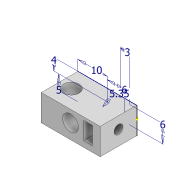
# Autodesk Inventor part: CentralStabalizerShaft
Saved by Autodesk Inventor 2022 (Build 260153000, 153)
## iProperties
Created: 2022-10-26
Part Number: CentralStabalizerShaft
Material: Generic
Document SubType Name: Modeling
Designer: MVeszpremi
Density: 1 g/cm^3
Appearance: Default
Author: MVeszpremi
Autodesk Inventor part; units mm, degrees
ref_plane "YZ Plane" through (0, 0, 0) normal (1, 0, 0) x (0, 1, 0)
ref_plane "XZ Plane" through (0, 0, 0) normal (0, 1, 0) x (-1, 0, 0)
ref_plane "XY Plane" through (0, 0, 0) normal (0, 0, 1) x (1, 0, 0)
sketch "Sketch1" plane through (0, 0, 0) normal (0, 0, 1) x (1, 0, 0)
  circle A0 centre (0, 0) radius 2.675
  line L0 (-10, 4) -> (10.0805, 4)
  line L1 (10.0805, 4) -> (10.0805, -5)
  line L2 (10.0805, -5) -> (-10, -5)
  line L3 (-10, -5) -> (-10, 4)
  line L4 (7.5, -3) -> (4.5, -3)
  line L5 (4.5, -3) -> (4.5, 3)
  line L6 (4.5, 3) -> (7.5, 3)
  line L7 (7.5, 3) -> (7.5, -3)
  line L8 (7.5, -3) -> (4.5, 3) construction
  line L9 (4.5, -3) -> (7.5, 3) construction
  point P0 (6, 0)
  dimension "d0" = 5.35
  dimension "d1" = 4
  dimension "d2" = 5
  dimension "d3" = 10
  dimension "d4" = 3
  dimension "d5" = 6
  dimension "d6" = 6
  constraints: 20 end point, 4 parallel, 2 horizontal, 2 midpoint, 2 perpendicular, 1 centre point, 1 coincident
  measures "d0" diameter of A0
  measures "d1" distance from line of L0 point (0, 0)
  measures "d2" distance from line of L2 point (0, 0)
  measures "d3" distance from line of point (0, 0) L3
  measures "d4" distance of L5.end L6.end
  measures "d5" distance of L6.end L4.start
  measures "d6" distance of point (6, 0) point (0, 0)
extrude "Extrusion1" add sketch "Sketch1" along normal blind 12.5
sketch "Sketch2" plane through (10.0805, -5, 0) normal (1, 0, 0) x (0, 0, -1)
  point P0 (0, 5)
sketch "Sketch3" plane through (10.0805, -5, 0) normal (1, 0, 0) x (0, 0, -1)
  line L0 (-12.5, 2.325) -> (0, 2.325) projected
  line L1 (-12.5, 2.325) -> (0, 7.675)
  line L2 (-12.5, 7.675) -> (0, 7.675) projected
  circle A0 centre (-6.25, 5) radius 1.5
  point P0 (0, 5)
  dimension "d9" = 3
  constraints: 2 end point, 2 point on line, 1 centre point, 1 midpoint
  measures "d9" diameter of A0
extrude "Extrusion2" cut sketch "Sketch3" against normal blind 10.25
sketch "Sketch4" plane through (-10, 4, 0) normal (0, 1, 0) x (1, 0, 0)
  circle A0 centre (4, -6.25) radius 2.675
  line L0 (0, 0) -> (0, -12.5) projected
  point P0 (10, 0)
  dimension "d12" = 5.35
  dimension "d13" = 4
  constraints: 1 centre point
  measures "d12" diameter of A0
  measures "d13" distance from line of L0 A0.centre
extrude "Extrusion3" cut sketch "Sketch4" against normal blind 14
body "Solid1"
